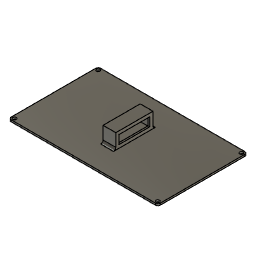
nts1-back v2 (Autodesk Fusion 360 design; units mm, degrees)
Autodesk Fusion 360 part; units mm, degrees
sketch "Sketch1" plane through (0, 0, 0) normal (0, 0, 1) x (1, 0, 0)
  line L0 (2, 0) -> (126.5, 0)
  line L1 (128.5, 2) -> (128.5, 75)
  line L2 (126.5, 77) -> (2, 77)
  line L3 (0, 75) -> (0, 2)
  line L4 (0, 74.5) -> (128.5, 74.5) construction
  line L5 (0, 2.5) -> (128.5, 2.5) construction
  line L6 (126, 77) -> (126, 0) construction
  line L7 (2.5, 77) -> (2.5, 0) construction
  circle A0 centre (2.5, 74.5) radius 1.5
  circle A1 centre (126, 74.5) radius 1.5
  circle A2 centre (126, 2.5) radius 1.5
  circle A3 centre (2.5, 2.5) radius 1.5
  arc A4 (2, 77) -> (0, 75) centre (2, 75) ccw
  arc A5 (128.5, 75) -> (126.5, 77) centre (126.5, 75) ccw
  arc A6 (126.5, 0) -> (128.5, 2) centre (126.5, 2) ccw
  arc A7 (0, 2) -> (2, 0) centre (2, 2) ccw
  point P0 (128.5, 0)
  point P1 (0, 77)
  dimension "d1" = 128.5
  dimension "d2" = 77
  dimension "d4" = 3
  dimension "d5" = 3
  dimension "d6" = 3
  dimension "d7" = 3
  dimension "d8" = 2.5
  dimension "d9" = 2.5
  dimension "d10" = 2.5
  dimension "d11" = 2.5
  dimension "d12" = 2
  dimension "d13" = 2
  dimension "d14" = 2
  dimension "d15" = 2
  constraint horizontal L0
  constraint vertical L1
  constraint horizontal L2
  constraint vertical L3
  constraint coincident L3 L4.start
  constraint perpendicular L3 L4
  constraint coincident L1 L4.end
  constraint coincident L3 L5.start
  constraint perpendicular L3 L5
  constraint coincident L1 L5.end
  constraint coincident L2 L6.start
  constraint perpendicular L2 L6
  constraint coincident L0 L6.end
  constraint coincident L2 L7.start
  constraint perpendicular L2 L7
  constraint coincident L0 L7.end
  constraint coincident L7 A0.centre
  constraint coincident L4 A0.centre
  constraint coincident L4 A1.centre
  constraint coincident L6 A1.centre
  constraint coincident L5 A2.centre
  constraint coincident L6 A2.centre
  constraint coincident L5 A3.centre
  constraint coincident L7 A3.centre
  constraint coincident P1 L2
  constraint coincident P1 L3
  constraint tangent L2 A4
  constraint tangent L3 A4
  constraint tangent L2 A5
  constraint tangent L1 A5
  constraint coincident P0 L1
  constraint coincident P0 L0
  constraint tangent L1 A6
  constraint tangent L0 A6
  constraint coincident origin L3
  constraint coincident origin L0
  constraint tangent L3 A7
  constraint tangent L0 A7
  measures "d1" distance of origin P0
  measures "d2" distance of origin P1
  measures "d4" diameter of A0
  measures "d5" diameter of A1
  measures "d6" diameter of A2
  measures "d7" diameter of A3
  measures "d8" distance of L2 L4
  measures "d9" distance of L3 L7
  measures "d10" distance of L1 L6
  measures "d11" distance of L0 L5
  measures "d12" radius of A4
  measures "d13" radius of A5
  measures "d14" radius of A6
  measures "d15" radius of A7
extrude "Extrude1" add sketch "Sketch1" along normal blind 1.5
sketch "Sketch2" plane through (0, 0, 1.5) normal (0, 0, 1) x (-1, 0, 0)
  circle A0 centre (-2.5, -74.5) radius 1.5
  circle A1 centre (-2.5, -2.5) radius 1.5
  circle A2 centre (-126, -2.5) radius 1.5
  circle A3 centre (-126, -74.5) radius 1.5
  arc A4 (0, -2) -> (-2, 0) centre (-2, -2) ccw
  line L0 (-2, 0) -> (-126.5, 0)
  arc A5 (-126.5, 0) -> (-128.5, -2) centre (-126.5, -2) ccw
  line L1 (-128.5, -2) -> (-128.5, -75)
  arc A6 (-128.5, -75) -> (-126.5, -77) centre (-126.5, -75) ccw
  line L2 (-126.5, -77) -> (-2, -77)
  arc A7 (-2, -77) -> (0, -75) centre (-2, -75) ccw
  line L3 (0, -75) -> (0, -2)
  line L4 (0, -38.5) -> (-128.5, -38.5) construction
  line L5 (-64.25, -77) -> (-64.25, 0) construction
  line L6 (-58.75, -22.5) -> (-69.75, -22.5)
  line L7 (-69.75, -22.5) -> (-69.75, -54.5)
  line L8 (-69.75, -54.5) -> (-58.75, -54.5)
  line L9 (-58.75, -54.5) -> (-58.75, -22.5)
  line L10 (-58.75, -22.5) -> (-69.75, -54.5) construction
  line L11 (-69.75, -22.5) -> (-58.75, -54.5) construction
  point P0 (-64.25, -38.5)
  dimension "d18" = 11
  dimension "d19" = 32
  constraint midpoint L3 L4.start
  constraint midpoint L1 L4.end
  constraint midpoint L2 L5.start
  constraint midpoint L0 L5.end
  constraint horizontal L6
  constraint perpendicular L6 L7
  constraint parallel L6 L8
  constraint parallel L7 L9
  constraint coincident L10 P0
  constraint coincident L11 P0
  constraint midpoint L4 P0
  measures "d18" distance of L7.end L8.end
  measures "d19" distance of L6.end L7.end
extrude "Extrude2" add sketch "Sketch2" along normal blind 13 contours L6 L7 L8 L9
sketch "Sketch3" plane through (58.75, 0, 0) normal (-1, 0, 0) x (0, -1, 0)
  line L0 (-54.5, 1.5) -> (-22.5, 1.5)
  line L1 (-22.5, 1.5) -> (-22.5, 14.5)
  line L2 (-22.5, 14.5) -> (-54.5, 14.5)
  line L3 (-54.5, 14.5) -> (-54.5, 1.5)
  line L4 (-54.5, 8) -> (-22.5, 8) construction
  line L5 (-38.5, 14.5) -> (-38.5, 1.5) construction
  line L6 (-24.25, 3) -> (-52.75, 3)
  line L7 (-52.75, 3) -> (-52.75, 13)
  line L8 (-52.75, 13) -> (-24.25, 13)
  line L9 (-24.25, 13) -> (-24.25, 3)
  line L10 (-24.25, 3) -> (-52.75, 13) construction
  line L11 (-52.75, 3) -> (-24.25, 13) construction
  line L12 (-25.25, 11.75) -> (-51.75, 11.75)
  line L13 (-51.75, 11.75) -> (-51.75, 4.25)
  line L14 (-51.75, 4.25) -> (-25.25, 4.25)
  line L15 (-25.25, 4.25) -> (-25.25, 11.75)
  line L16 (-25.25, 11.75) -> (-51.75, 4.25) construction
  line L17 (-51.75, 11.75) -> (-25.25, 4.25) construction
  point P0 (-38.5, 8)
  point P1 (-38.5, 8)
  dimension "d22" = 28.5
  dimension "d23" = 10
  dimension "d24" = 26.5
  dimension "d25" = 7.5
  constraint midpoint L3 L4.start
  constraint midpoint L1 L4.end
  constraint midpoint L2 L5.start
  constraint midpoint L0 L5.end
  constraint horizontal L6
  constraint perpendicular L6 L7
  constraint parallel L6 L8
  constraint parallel L7 L9
  constraint coincident L10 P1
  constraint coincident L11 P1
  constraint midpoint L4 P1
  constraint horizontal L12
  constraint perpendicular L12 L13
  constraint parallel L12 L14
  constraint parallel L13 L15
  constraint coincident L16 P1
  constraint coincident L17 P1
  constraint coincident P1 P0
  measures "d22" distance of L7.end L8.end
  measures "d23" distance of L6.end L7.end
  measures "d24" distance of L13.end L14.end
  measures "d25" distance of L12.end L13.end
extrude "Extrude3" cut sketch "Sketch3" against normal blind 30 contours L12 L13 L14 L15
extrude "Extrude4" cut sketch "Sketch3" against normal blind 9.5 contours L6 L7 L8 L9
fillet "Fillet1" radius 2 1 edges at (64.25, 22.5, 1.5)
fillet "Fillet2" radius 2 1 edges at (64.25, 54.5, 1.5)
equation "mounting_hole = 3 mm"
equation "d4 = mounting_hole"
equation "d5 = mounting_hole"
equation "d6 = mounting_hole"
equation "d7 = mounting_hole"
